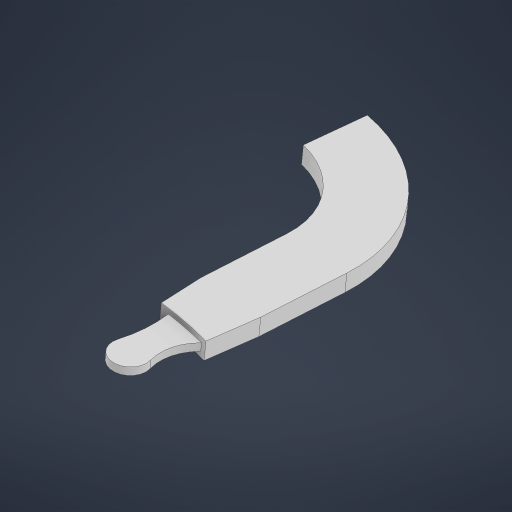
# Autodesk Inventor part: long
Saved by Autodesk Inventor 2024 (Build 280153000, 153)
## iProperties
Created: 2024-12-18
Part Number: long
Material: Generic
Document SubType Name: Modeling
Designer: Alex
Density: 1 g/cm^3
Appearance: Default
Author: Alex
Autodesk Inventor part; units mm, degrees
sketch "Sketch1" plane through (0, 0, 0) normal (0, 1, 0) x (-1, 0, 0)
  circle A0 centre (0, 0) radius 10
  line L0 (10, 0) -> (9.2097, -30.1236) construction
  arc A1 (-17.027, -27.0939) -> (14.3169, -30.2866) centre (17.8178, 159.5407) ccw
  line L1 (0, 0) -> (-14.0737, -27.6212) construction
  line L2 (10, 0) -> (-10, 0) construction
  line L3 (0, -10) -> (0, 10) construction
  arc A2 (9.7489, -2.227) -> (9.2097, -30.1236) centre (76.4766, -17.4702) ccw
  arc A3 (-14.0737, -27.6212) -> (-9.4804, -3.1816) centre (-33.645, -11.2914) ccw
  line L4 (0, 0) -> (9.2097, -30.1236) construction
  line L5 (14.3169, -30.2866) -> (-17.027, -27.0939) construction
  line L6 (9.2097, -30.1236) -> (-14.0737, -27.6212) construction
  line L7 (-1.355, -28.6902) -> (-1.4214, -29.3415) construction
  line L8 (0, 0) -> (-17.027, -27.0939) construction
  line L9 (0, 0) -> (14.3169, -30.2866) construction
  line L10 (-17.027, -27.0939) -> (-14.0737, -27.6212) construction
  line L11 (0, 0) -> (-18.5691, -57.0543) construction
  line L12 (0, 0) -> (17.8587, -58.3272) construction
  line L13 (17.8587, -58.3272) -> (-18.5691, -57.0543) construction
  line L14 (-18.5691, -57.0543) -> (-17.027, -27.0939) construction
  line L15 (14.3169, -30.2866) -> (17.8587, -58.3272) construction
  line L16 (14.3169, -30.2866) -> (17.8587, -58.3272)
  line L17 (-17.027, -27.0939) -> (-18.5691, -57.0543)
  line L18 (17.8587, -58.3272) -> (31.4475, -86.1902) construction
  line L19 (-18.5691, -57.0543) -> (3.1581, -110.8309) construction
  line L20 (-18.5691, -57.0543) -> (39.4309, -57.0543) construction
  arc A4 (17.8587, -58.3272) -> (31.4475, -86.1902) centre (65.5771, -52.3) ccw
  arc A5 (-18.5691, -57.0543) -> (3.1581, -110.8309) centre (50.0978, -60.5886) ccw
  line L21 (31.4475, -86.1902) -> (3.1581, -110.8309)
  dimension "d0" = 20
  dimension "d4" = 63
  dimension "d7" = 31
  dimension "d8" = 73
  dimension "d9" = 31.5
  dimension "d14" = 32
  dimension "d15" = 33.5
  dimension "d19" = 3
  dimension "d20" = 60
  dimension "d21" = 61
  dimension "d22" = 36.45
  dimension "d23" = 30
  dimension "d24" = 68.4466
  dimension "d25" = 25.4892
  dimension "d26" = 118
  dimension "d27" = 31
  dimension "d28" = 58
  dimension "d29" = 68
  dimension "d30" = 37.5161
  constraints: 44 end point, 19 point on circle, 6 centre point, 4 tangent, 2 collinear, 2 horizontal, 1 coincident, 1 equal length, 1 midpoint, 1 vertical
  measures "d0" diameter of A0
  measures "d4" angle of L2 L1
  measures "d7" distance of L1.start L1.end
  measures "d8" angle of L2 L4
  measures "d9" distance of L1.start L0.end
  measures "d14" distance of L1.start L5.end
  measures "d15" distance of L1.start L5.start
  measures "d19" distance of L5.end L1.end
  measures "d20" distance of L1.start L11.end
  measures "d21" distance of L1.start L12.end
  measures "d22" distance of L12.end L11.end
  measures "d23" distance of L11.end L5.end
  measures "d24" radius of A2
  measures "d25" radius of A3
  measures "d26" angle of L13 L18
  measures "d27" distance of L12.end L18.end
  measures "d28" distance of L11.end L19.end
  measures "d29" angle of L19 L20
  measures "d30" distance of L18.end L19.end
ref_plane "Work Plane11" through (-31.4475, -5, -86.1902) normal (-0.6568, 0, -0.7541) x (-0.7541, 0, 0.6568)
sketch "Sketch2" plane through (-31.4475, -5, -86.1902) normal (-0.6568, 0, -0.7541) x (-0.7541, 0, 0.6568)
  line L0 (-18.5789, 0) -> (-18.5789, 10) construction
  line L1 (0, 0) -> (0, 10) construction
  line L2 (-37.5161, 10) -> (0, 10) construction
  line L3 (-37.5161, 0) -> (-37.5161, 10) construction
  line L4 (0, 0) -> (-37.5161, 0) construction
  line L5 (0, 5) -> (-37.5161, 5) construction
  point P0 (32.8968, 5)
  point P1 (-18.758, 5)
  constraints: 3 midpoint, 2 end point
ref_plane "Work Plane4" through (-31.4475, 0, -86.1902) normal (0, 1, 0) x (0.7541, 0, -0.6568)
ref_plane "Work Plane5" through (-31.4475, -148, -86.1902) normal (0, 1, 0) x (0.7541, 0, -0.6568)
sketch "Sketch3" plane through (-31.4475, -148, -86.1902) normal (0, 1, 0) x (0.7541, 0, -0.6568)
  line L0 (18.5789, -54.8214) -> (-2.262, -76.4005) projected
  point P0 (-32.8968, -85.6475)
ref_plane "Work Plane6" through (18.5691, -148, -57.0543) normal (0.057, 0.9984, 0.0029) x (-0.0514, 0, 0.9987)
sketch "Sketch4" plane through (18.5691, -148, -57.0543) normal (0.057, 0.9984, 0.0029) x (-0.0514, 0, 0.9987)
  line L0 (0, 0) -> (0, -25.972) construction
  point P0 (57.9333, -24.0285)
  constraints: 2 end point, 1 vertical
ref_plane "Work Plane7" through (18.5691, -148, -57.0543) normal (0.0596, 0.997, -0.0493) x (-0.9971, 0.057, -0.0513)
sketch "Sketch5" plane through (18.5691, -148, -57.0543) normal (0.0596, 0.997, -0.0493) x (-0.9971, 0.057, -0.0513)
  ellipse E0 centre (23.9002, 65.4229) end of major axis (30.6548, 58.0489) minor radius 9.97 construction
  circle A0 centre (23.9002, 65.4229) radius 10
  line L0 (31.314, 72.1337) -> (33.1099, 35.2993) construction
  arc A1 (6.8732, 38.3289) -> (38.2171, 35.1363) centre (41.718, 224.9636) ccw
  line L1 (23.9002, 65.4229) -> (9.8265, 37.8017) construction
  line L2 (31.314, 72.1337) -> (16.4863, 72.1337) construction
  arc A2 (33.649, 63.1959) -> (33.1099, 35.2993) centre (100.3768, 47.9527) ccw
  arc A3 (9.8265, 37.8017) -> (14.4198, 62.2412) centre (-9.7448, 54.1315) ccw
  line L3 (23.9002, 65.4229) -> (33.1099, 35.2993) construction
  line L4 (38.2171, 35.1363) -> (6.8732, 38.3289) construction
  line L5 (33.1099, 35.2993) -> (9.8265, 37.8017) construction
  line L6 (22.5451, 36.7326) -> (22.4788, 36.0813) construction
  line L7 (23.9002, 65.4229) -> (6.8732, 38.3289) construction
  line L8 (23.9002, 65.4229) -> (38.2171, 35.1363) construction
  line L9 (6.8732, 38.3289) -> (9.8265, 37.8017) construction
  line L10 (23.9002, 65.4229) -> (6.0481, 8.1402) construction
  line L11 (23.9002, 65.4229) -> (41.7677, 9.6133) construction
  line L12 (41.7677, 9.6133) -> (6.0481, 8.1402) construction
  line L13 (6.0481, 8.1402) -> (6.8732, 38.3289) construction
  line L14 (38.2171, 35.1363) -> (41.7677, 9.6133) construction
  line L15 (38.2171, 35.1363) -> (41.7677, 9.6133)
  line L16 (6.8732, 38.3289) -> (6.0481, 8.1402)
  line L17 (41.7677, 9.6133) -> (43.8485, -40.8438)
  line L18 (6.0481, 8.1402) -> (8.1289, -42.3169)
  line L19 (8.1289, -42.3169) -> (43.8485, -40.8438) construction
  line L20 (8.1289, -42.3169) -> (81.3932, -124.3678) construction
  line L21 (43.8485, -40.8438) -> (86.8081, -88.9555) construction
  arc A4 (8.1289, -42.3169) -> (81.3932, -124.3678) centre (94.7052, -38.7465) ccw
  arc A5 (43.8485, -40.8438) -> (86.8081, -88.9555) centre (94.6137, -38.7503) ccw
  line L22 (86.8081, -88.9555) -> (86.8081, -125.0358)
  arc A6 (81.3932, -124.3678) -> (86.8081, -125.0358) centre (94.7052, -38.7465) ccw
  point P0 (24.0285, 65.5404)
  point P1 (14.611, 61.7909)
  point P2 (33.7346, 63.6729)
  point P3 (33.532, 68.1115)
  point P4 (33.532, 68.1115)
  dimension "d41" = 20
  dimension "d42" = 63
  dimension "d43" = 31
  dimension "d44" = 73
  dimension "d45" = 31.5
  dimension "d46" = 32
  dimension "d47" = 33.5
  dimension "d48" = 3
  dimension "d49" = 60
  dimension "d50" = 58.6
  dimension "d51" = 35.75
  dimension "d52" = 30.2
  dimension "d53" = 68.4466
  dimension "d54" = 25.4892
  dimension "d60" = 50.5
  dimension "d62" = 50.5
  dimension "d63" = 110
  dimension "d64" = 64.5
  dimension "d65" = 85
  constraints: 46 end point, 21 point on circle, 7 centre point, 5 tangent, 3 coincident, 2 collinear, 2 parallel, 1 concentric, 1 horizontal, 1 midpoint, 1 perpendicular, 1 vertical, 3 other
  measures "d41" diameter of A0
  measures "d42" angle of L2 L1
  measures "d43" distance of L8.start L9.end
  measures "d44" angle of L2 L3
  measures "d45" distance of L8.start L5.start
  measures "d46" distance of L8.start L9.start
  measures "d47" distance of L8.start L8.end
  measures "d48" distance of L9.start L9.end
  measures "d49" distance of L8.start L10.end
  measures "d50" distance of L8.start L11.end
  measures "d51" distance of L11.end L10.end
  measures "d52" distance of L10.end L9.start
  measures "d53" radius of A2
  measures "d54" radius of A3
  measures "d60" distance of L11.end L17.end
  measures "d62" distance of L10.end L18.end
  measures "d63" distance of L18.end L20.end
  measures "d64" distance of L17.end L21.end
  measures "d65" distance from line of L19 L20.end
ref_plane "Work Plane9" through (-31.4475, -74, -86.1902) normal (0, 1, 0) x (0.7541, 0, -0.6568)
ref_plane "Work Plane10" through (6.9439, -145.4643, -19.8528) normal (0.057, 0.9984, 0.0029) x (-0.0514, 0, 0.9987)
sketch "Sketch6" plane through (6.9439, -145.4643, -19.8528) normal (0.057, 0.9984, 0.0029) x (-0.0514, 0, 0.9987)
  line L0 (-2.499, -23.2834) -> (0, 0) construction
  ellipse E0 centre (186.9054, -31.8915) end of major axis (186.9054, -221.7511) minor radius 189.5994 (0.5265, 2.9533) -> (-2.6617, -28.3906) ccw projected
  circle A0 centre (27.6212, -14.0737) radius 10
  line L1 (27.6224, -24.0737) -> (-2.5024, -23.2834) construction
  arc A1 (0.5273, 2.9533) -> (-2.6654, -28.3906) centre (187.1619, -31.8915) ccw
  line L2 (27.6212, -14.0737) -> (0, 0) construction
  line L3 (27.6224, -24.0737) -> (27.6224, -4.0737) construction
  line L4 (24.2804, -23.4992) -> (30.962, -23.4992) construction
  arc A2 (25.3942, -23.8226) -> (-2.5024, -23.2834) centre (10.151, -90.5503) ccw
  arc A3 (0, 0) -> (24.4396, -4.5934) centre (16.3298, 19.5713) ccw
  line L5 (27.6212, -14.0737) -> (-2.5024, -23.2834) construction
  line L6 (-2.6654, -28.3906) -> (0.5273, 2.9533) construction
  line L7 (-2.5024, -23.2834) -> (0, 0) construction
  line L8 (-1.069, -12.7187) -> (-1.7203, -12.6523) construction
  line L9 (27.6212, -14.0737) -> (0.5273, 2.9533) construction
  line L10 (27.6212, -14.0737) -> (-2.6654, -28.3906) construction
  line L11 (0.5273, 2.9533) -> (0, 0) construction
  point P0 (20.1835, -14.202)
  point P1 (-2.4989, -23.2828)
  dimension "d66" = 20
  dimension "d67" = 63
  dimension "d68" = 31
  dimension "d69" = 73
  dimension "d70" = 31.5
  dimension "d71" = 32
  dimension "d72" = 33.5
  dimension "d73" = 3
  dimension "d74" = 68.4466
  dimension "d75" = 25.4892
  dimension "d83" = 85.377
  dimension "d84" = 8.3924
  dimension "d85" = 0
  dimension "d86" = 30.1213
  constraints: 22 end point, 15 point on circle, 4 centre point, 2 tangent, 1 coincident, 1 horizontal, 1 midpoint, 1 vertical, 1 other
  measures "d66" diameter of A0
  measures "d67" angle of L3 L2
  measures "d68" distance of L0.end L2.start
  measures "d69" angle of L3 L5
  measures "d70" distance of L2.start L5.end
  measures "d71" distance of L2.start L9.end
  measures "d72" distance of L2.start L10.end
  measures "d73" distance of L0.end L9.end
  measures "d74" radius of A2
  measures "d75" radius of A3
  measures "d83" angle of L0 L1
  measures "d84" distance from line of point (186.905, -31.892) L4
  measures "d85" distance from line of point (-2.499, -23.283) L0
  measures "d86" distance from line of point (-2.499, -23.283) L3
extrude "Extrusion4" add sketch "Sketch6" along normal mid plane 4.5
extrude "Extrusion5" add sketch "Sketch5" along normal mid plane 10 contours A1 L15 L17 A5 L22 A6 A4 L18 L16
body "Solid1"
